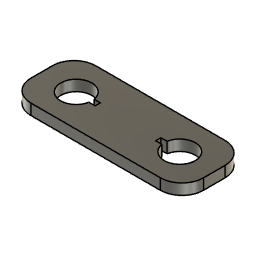
Top plate v1 (Autodesk Fusion 360 design; units mm, degrees)
Autodesk Fusion 360 part; units mm, degrees
sketch "Sketch1" plane through (0, 0, 0) normal (0, 0, 1) x (1, 0, 0)
  line L0 (0, 0) -> (40, 0)
  line L1 (40, 0) -> (40, 15)
  line L2 (40, 15) -> (0, 15)
  line L3 (0, 15) -> (0, 0)
  dimension "d1" = 40
  dimension "d2" = 15
  constraint horizontal L0
  constraint vertical L1
  constraint horizontal L2
  constraint vertical L3
  constraint coincident L0.start L3.end
  measures "d1" distance of L0.start L0.end
  measures "d2" distance of L0.start L2.end
extrude "Extrude1" add sketch "Sketch1" along normal blind 2.5
sketch "Sketch2" plane through (0, 0, 2.5) normal (0, 0, 1) x (-1, 0, 0)
  line L0 (0, -15) -> (0, 0)
  line L1 (0, 0) -> (-40, 0)
  line L2 (-40, 0) -> (-40, -15)
  line L3 (-40, -15) -> (0, -15)
  line L4 (-20, -20) -> (-20, 7) construction
  line L5 (-32, -20) -> (-32, 13) construction
  line L6 (-8, -20) -> (-8, 12) construction
  line L7 (2.5927, -7.5) -> (-48, -7.5) construction
  line L8 (-13, -8.1) -> (-13, -6.9)
  line L9 (-27, -8.1) -> (-27, -6.9)
  arc A0 (-11.5496, -8.1) -> (-11.5496, -6.9) centre (-8, -7.5) ccw
  line L10 (-28.4504, -6.9) -> (-27, -6.9)
  line L11 (-13, -6.9) -> (-11.5496, -6.9)
  line L12 (-11.5496, -8.1) -> (-13, -8.1)
  line L13 (-27, -8.1) -> (-28.4504, -8.1)
  arc A1 (-28.4504, -6.9) -> (-28.4504, -8.1) centre (-32, -7.5) ccw
  dimension "d5" = 20
  dimension "d6" = 12
  dimension "d7" = 12
  dimension "d8" = 7.5
  dimension "d9" = 7.2
  dimension "d10" = 7.2
  dimension "d12" = 0.6
  dimension "d13" = 5
  dimension "d14" = 5
  constraint vertical L4
  constraint perpendicular L3 L5
  constraint vertical L6
  constraint perpendicular L2 L7
  constraint coincident L7 A1.centre
  constraint coincident L5 A1.centre
  constraint coincident L7 A0.centre
  constraint coincident L6 A0.centre
  constraint horizontal L12
  constraint horizontal L10
  constraint perpendicular L8 L12
  constraint perpendicular L7 L9
  constraint coincident L8.end L10
  constraint collinear L10 L11
  constraint collinear L12 L13
  measures "d5" distance of L2 L4
  measures "d6" distance of L4 L5
  measures "d7" distance of L4 L6
  measures "d8" distance of L3 L7
  measures "d9" diameter of A1
  measures "d10" diameter of A0
  measures "d12" distance of L7 L12
  measures "d13" distance of A0.centre L8
  measures "d14" distance of A1.centre L9
extrude "Extrude2" cut sketch "Sketch2" against normal blind 4 contours L8 A0 L11 L12 | L9 L10 L13 A1
fillet "Fillet1" radius 5 1 edges at (0, 0, 1.25)
fillet "Fillet2" radius 5 2 edges at (40, 0, 1.25) (40, 15, 1.25)
fillet "Fillet3" radius 5 1 edges at (0, 15, 1.25)
